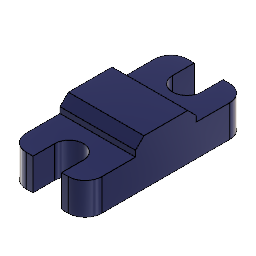
1-Belt-clamp_1 (Autodesk Fusion 360 design; units mm, degrees)
Autodesk Fusion 360 part; units mm, degrees
imported_body "Base Feature1" makes body 1
sketch "Sketch1" plane through (0, 0, 0) normal (0, 0, 1) x (1, 0, 0)
  line L0 (4.5, 9.6) -> (-4.5, 9.6)
  line L1 (-4.5, 9.6) -> (-4.5, -9.6)
  line L2 (-4.5, -9.6) -> (4.5, -9.6)
  line L3 (4.5, -9.6) -> (4.5, 9.6)
  line L4 (4.5, 9.6) -> (-4.5, -9.6) construction
  line L5 (-4.5, 9.6) -> (4.5, -9.6) construction
  line L6 (-1.7, -9.6) -> (-1.7, -7)
  line L7 (1.7, -9.6) -> (1.7, -7)
  arc A0 (1.7, -7) -> (-1.7, -7) centre (0, -7) ccw
  line L8 (1.75, 0) -> (22.5, 0)
  line L9 (-1.7, 9.6) -> (-1.7, 7)
  arc A1 (-1.7, 7) -> (1.7, 7) centre (0, 7) ccw
  line L10 (1.7, 9.6) -> (1.7, 7)
  line L11 (4.5, -3.6) -> (-4.5, -3.6)
  line L12 (-4.5, -3.6) -> (-4.5, 3.6)
  line L13 (-4.5, 3.6) -> (4.5, 3.6)
  line L14 (4.5, 3.6) -> (4.5, -3.6)
  line L15 (0, 0) -> (-4.5, 0) construction
  dimension "d1" = 9
  dimension "d2" = 19.2
  dimension "d3" = 3.4
  dimension "d4" = 2.6
  dimension "d5" = 7.2
  measures "d3" distance of L6 L7
  measures "d4" distance of L2
  measures "d5" distance of L11 L13
extrude "Extrude1" add sketch "Sketch1" along normal blind 3.8 separate body contours L0 L1 L3 L9 A1 L10 L13 | L1 L3 L11 L12 L13 L14 | L1 L2 L3 L6 L7 A0 L11 makes body 2
extrude "Extrude2" add sketch "Sketch1" along normal blind 1.7 from surface at 3.8 contours L1 L3 L11 L12 L13 L14 bodies 2
chamfer "Chamfer1" distance 1 angle 45 2 edges at (0, -3.6, 5.5) (0, 3.6, 5.5) on bodies 2
fillet "Fillet1" radius 2 4 edges at (-4.5, -9.6, 1.9) (4.5, -9.6, 1.9) (4.5, 9.6, 1.9) (-4.5, 9.6, 1.9) on bodies 2
hidden bodies 1
